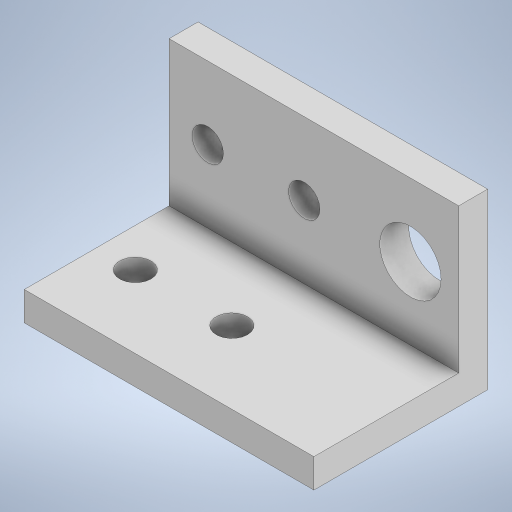
# Autodesk Inventor part: Base_Connector1
Saved by Autodesk Inventor 2023 (Build 270158000, 158)
## iProperties
Created: 2023-02-08
Part Number: Base_Connector1
Material: Generic
Document SubType Name: Modeling
Designer: deepa
Density: 1 g/cm^3
Appearance: Default
Author: deepa
Autodesk Inventor part; units mm, degrees
ref_plane "YZ Plane" through (0, 0, 0) normal (1, 0, 0) x (0, 1, 0)
ref_plane "XZ Plane" through (0, 0, 0) normal (0, 1, 0) x (-1, 0, 0)
ref_plane "XY Plane" through (0, 0, 0) normal (0, 0, 1) x (1, 0, 0)
sketch "Sketch1" plane through (0, 0, 0) normal (1, 0, 0) x (0, 1, 0)
  line L0 (0, 0) -> (0, 36)
  line L1 (0, 36) -> (6, 36)
  line L2 (6, 36) -> (6, 6)
  line L3 (6, 6) -> (36, 6)
  line L4 (36, 6) -> (36, 0)
  line L5 (36, 0) -> (0, 0)
  dimension "d0" = 36
  dimension "d1" = 6
  dimension "d2" = 30
  dimension "d3" = 30
  dimension "d4" = 6
  dimension "d5" = 36
  constraints: 12 end point, 4 perpendicular, 1 vertical
  measures "d0" distance of L0.start L0.end
  measures "d1" distance of L0.end L1.end
  measures "d2" distance of L1.end L2.end
  measures "d3" distance of L2.end L3.end
  measures "d4" distance of L3.end L4.end
  measures "d5" distance of L4.end L0.start
extrude "Extrusion1" add sketch "Sketch1" against normal blind 60
sketch "Sketch2" plane through (0, 6, 36) normal (0, 1, 0) x (1, 0, 0)
  circle A0 centre (-52, 15) radius 3.25
  circle A1 centre (-32, 15) radius 3.25
  line L0 (0, 0) -> (-60, 0) projected
  line L1 (0, 30) -> (0, 0) projected
  line L2 (-60, 0) -> (-60, 30) projected
  line L3 (-60, 30) -> (-20.277, 30) construction
  point P0 (0, 36)
  point P1 (-5.4498, 30)
  dimension "d8" = 6.5
  dimension "d9" = 6.5
  dimension "d10" = 20
  dimension "d11" = 15
  dimension "d12" = 15
  dimension "d13" = 32
  constraints: 2 centre point, 2 end point, 1 coincident, 1 horizontal
  measures "d8" diameter of A0
  measures "d9" diameter of A1
  measures "d10" distance of A1.centre A0.centre
  measures "d11" distance from line of L0 A1.centre
  measures "d12" distance from line of L0 A0.centre
  measures "d13" distance from line of L1 A1.centre
sketch "Sketch3" plane through (0, 6, 6) normal (0, 0, 1) x (1, 0, 0)
  circle A0 centre (-52, 15) radius 3.25
  line L0 (-60, 0) -> (-60, 30) projected
  line L1 (0, 30) -> (-60, 30) projected
  circle A1 centre (-32, 15) radius 3.25
  point P0 (0, -6)
  dimension "d14" = 6.5
  dimension "d15" = 8
  dimension "d16" = 15
  dimension "d17" = 6.5
  dimension "d18" = 20
  constraints: 2 centre point
  measures "d14" diameter of A0
  measures "d15" distance from line of L0 A0.centre
  measures "d16" distance from line of L1 A0.centre
  measures "d17" diameter of A1
  measures "d18" distance of A1.centre A0.centre
extrude "Extrusion2" cut sketch "Sketch3" against normal blind 6
extrude "Extrusion3" cut sketch "Sketch2" against normal blind 6
sketch "Sketch4" plane through (0, 6, 6) normal (0, 0, 1) x (1, 0, 0)
  circle A0 centre (-10, 15) radius 6.35
  line L0 (0, 30) -> (0, 0) projected
  point P0 (0, -6)
  point P1 (0, 15)
  dimension "d23" = 12.7
  dimension "d24" = 10
  constraints: 1 centre point, 1 midpoint
  measures "d23" diameter of A0
  measures "d24" distance of A0.centre point (0, 15)
extrude "Extrusion4" cut sketch "Sketch4" against normal blind 6
body "Solid1"
